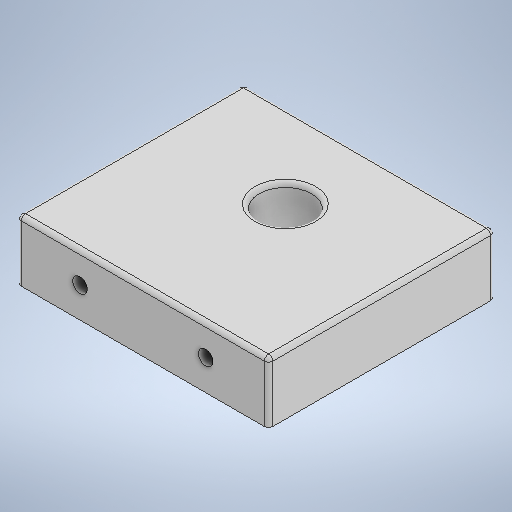
# Autodesk Inventor part: dessus_cadre
Saved by Autodesk Inventor 2025.1 (Build 291241000, 241)
## iProperties
Created: 2025-05-14
Part Number: dessus_cadre
Material: Générique
Document SubType Name: Modeling
Designer: chapuzet
Density: 1 g/cm^3
Appearance: Par défaut
Author: chapuzet
Autodesk Inventor part; units mm, degrees
ref_plane "YZ Plane" through (0, 0, 0) normal (1, 0, 0) x (0, 1, 0)
ref_plane "XZ Plane" through (0, 0, 0) normal (0, 1, 0) x (-1, 0, 0)
ref_plane "XY Plane" through (0, 0, 0) normal (0, 0, 1) x (1, 0, 0)
sketch "Esquisse1" plane through (0, 0, 0) normal (0, 1, 0) x (-1, 0, 0)
  line L0 (-30, 27) -> (30, 27)
  line L1 (30, 27) -> (30, -27)
  line L2 (30, -27) -> (-30, -27)
  line L3 (-30, -27) -> (-30, 27)
  line L4 (-30, 27) -> (30, -27) construction
  line L5 (30, 27) -> (-30, -27) construction
  circle A0 centre (0, -7) radius 6.25
  point P0 (0, 0)
  dimension "d0" = 54
  dimension "d1" = 60
  dimension "d2" = 34
  dimension "d3" = 12.5
  constraints: 12 end point, 2 midpoint, 2 parallel, 1 centre point, 1 horizontal, 1 perpendicular
  measures "d0" distance of L0.end L1.end
  measures "d1" distance of L1.end L2.end
  measures "d2" distance from line of L0 A0.centre
  measures "d3" diameter of A0
extrude "Extrusion1" add sketch "Esquisse1" along normal blind 14.5
sketch "Esquisse2" plane through (-30, 0, 27) normal (0, 0, 1) x (1, 0, 0)
  line L0 (0, 0) -> (0, 14.5) projected
  line L1 (60, 0) -> (0, 0) projected
  line L2 (0, 14.5) -> (60, 14.5)
  line L3 (60, 14.5) -> (60, 0)
  line L4 (60, 0) -> (0, 0)
  line L5 (0, 0) -> (0, 14.5)
  line L6 (0, 7.25) -> (60, 7.25)
  circle A0 centre (15, 7.25) radius 1.75
  circle A1 centre (45, 7.25) radius 1.75
  point P0 (30, 0)
  dimension "d6" = 15
  dimension "d7" = 15
  dimension "d8" = 3.5
  constraints: 10 end point, 2 centre point, 2 midpoint, 2 parallel, 2 point on line, 1 equal radius, 1 horizontal, 1 perpendicular
  measures "d6" distance from line of L3 A1.centre
  measures "d7" distance from line of L0 A0.centre
  measures "d8" diameter of A0
fillet "Congé1" radius 1 9 edges at (-30, 14.5, 0) (0, 14.5, -27) (30, 14.5, 0) (0, 14.5, 27) (30, 7.25, 27) (-30, 7.25, 27) (-30, 7.25, -27) (30, 7.25, -27) (6.25, 14.5, -7)
extrude "Extrusion2" cut sketch "Esquisse2" against normal blind 10 contours A0 L6 | L6 A0 | A1 L6 | L6 A1
